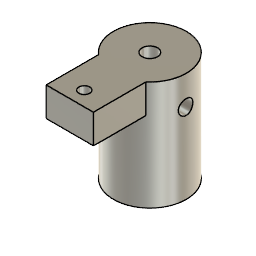
Lever Arm Potentiometer Coupler v9 (Autodesk Fusion 360 design; units mm, degrees)
Autodesk Fusion 360 part; units mm, degrees
sketch "Sketch1" plane through (0, 0, 0) normal (0, 0, 1) x (1, 0, 0)
  circle A0 centre (0, 0) radius 3.125
  circle A1 centre (0, 0) radius 10
  dimension "d1" = 6.25
  dimension "d2" = 20
  constraint coincident A0.centre A1.centre
  constraint concentric A0 A1
  measures "d1" diameter of A0
  measures "d2" diameter of A1
extrude "Extrude1" add sketch "Sketch1" along normal blind 15
sketch "Sketch7" plane through (0, 0, 15) normal (0, 0, 1) x (-1, 0, 0)
  circle A0 centre (0, 0) radius 3.125
  circle A1 centre (0, 0) radius 10
  circle A2 centre (0, 0) radius 2.125
  dimension "d28" = 4.25
  constraint concentric A0 A2
  measures "d28" diameter of A2
extrude "Extrude8" add sketch "Sketch7" along normal blind 15 contours A0 | A1
sketch "Sketch3" plane through (0, 0, 0) normal (1, 0, 0) x (0, 1, 0)
  circle A0 centre (0, 22) radius 2
  dimension "d20" = 4
  dimension "d21" = 22
  measures "d20" diameter of A0
  measures "d21" distance of origin A0.centre
extrude "Extrude3" cut sketch "Sketch3" along normal mid plane 20
sketch "Sketch8" plane through (0, 0, 0) normal (0, 1, 0) x (1, 0, 0)
  line L0 (-6.5, -22) -> (6.5, -22)
  line L1 (6.5, -22) -> (6.5, -30)
  line L2 (6.5, -30) -> (-6.5, -30)
  line L3 (-6.5, -30) -> (-6.5, -22)
  dimension "d31" = 13
  dimension "d32" = 8
  dimension "d33" = 30
  dimension "d36" = 6.5
  constraint horizontal L0
  constraint vertical L1
  constraint horizontal L2
  constraint vertical L3
  measures "d31" distance of L1 L3
  measures "d32" distance of L0 L2
  measures "d33" distance of origin L2
  measures "d36" distance of origin L1
extrude "Extrude9" add sketch "Sketch8" against normal blind 15 from surface at -7
sketch "Sketch10" plane through (0, 0, 30) normal (0, 0, 1) x (-1, 0, 0)
  arc A0 (-6.5, 7.5993) -> (6.5, 7.5993) centre (0, 0) ccw
  line L0 (6.5, 7.5993) -> (6.5, 22)
  line L1 (6.5, 22) -> (-6.5, 22)
  line L2 (-6.5, 22) -> (-6.5, 7.5993)
  circle A1 centre (0, 18) radius 1.5
  circle A2 centre (0, 0) radius 2.125
  dimension "d43" = 3
  dimension "d44" = 4
  dimension "d45" = 6.5
  measures "d43" diameter of A1
  measures "d44" distance of L1 A1.centre
  measures "d45" distance of L2 A1.centre
extrude "Extrude11" cut sketch "Sketch10" against normal blind 8 contours A1
sketch "Sketch11" plane through (0, 0, 0) normal (0, 0, -1) x (1, 0, 0)
  circle A0 centre (0, 0) radius 3.125
  circle A1 centre (0, 0) radius 10
  line L0 (-0.5, -4) -> (0.5, -4)
  line L1 (0.5, -4) -> (0.5, 4)
  line L2 (0.5, 4) -> (-0.5, 4)
  line L3 (-0.5, 4) -> (-0.5, -4)
  dimension "d48" = 1
  dimension "d49" = 0.5
  dimension "d50" = 8
  dimension "d51" = 4
  constraint horizontal L0
  constraint vertical L1
  constraint horizontal L2
  constraint vertical L3
  measures "d48" distance of L1 L3
  measures "d49" distance of A0.centre L3
  measures "d50" distance of L0 L2
  measures "d51" distance of A0.centre L0
extrude "Extrude12" add sketch "Sketch11" against normal blind 15 contours A0 L1 L3 | A0 L1 L2 L3 | A0 L0 L1 L3
